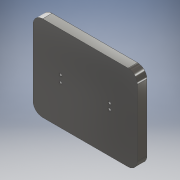
# Autodesk Inventor part: reverse gear stand
Saved by Autodesk Inventor 2017 (Build 210142000, 142)
## iProperties
Created: 2018-11-06
Part Number: reverse gear stand
Material: Generic
Document SubType Name: Modeling
Designer: User
Density: 1 g/cm^3
Appearance: Default
Author: User
Autodesk Inventor part; units mm, degrees
ref_plane "YZ Plane" through (0, 0, 0) normal (1, 0, 0) x (0, 1, 0)
ref_plane "XZ Plane" through (0, 0, 0) normal (0, 1, 0) x (-1, 0, 0)
ref_plane "XY Plane" through (0, 0, 0) normal (0, 0, 1) x (1, 0, 0)
sketch "Sketch2" plane through (0, 0, 0) normal (0, 1, 0) x (-1, 0, 0)
  line L0 (0, 0) -> (-220, 0)
  line L1 (-220, 0) -> (-220, -180)
  line L2 (-220, -180) -> (0, -180)
  line L3 (0, -180) -> (0, 0)
  dimension "d0" = 220
  dimension "d1" = 180
  constraints: 8 end point, 2 parallel, 1 horizontal, 1 perpendicular
  measures "d0" distance of L2.end L1.end
  measures "d1" distance of L1.end L0.end
extrude "Extrusion1" add sketch "Sketch2" along normal blind 20
sketch "Sketch3" plane through (0, 20, 0) normal (0, 1, 0) x (1, 0, 0)
  line L0 (0, 20) -> (0, 160)
  line L1 (0, 90) -> (46.5, 90)
  line L2 (46.5, 90) -> (173.5, 90)
  line L3 (173.5, 90) -> (173.5, 109)
  line L4 (173.5, 109) -> (173.5, 71)
  line L5 (173.5, 71) -> (46.5, 71)
  line L6 (46.5, 71) -> (46.5, 109)
  line L7 (46.5, 109) -> (173.5, 109)
  line L8 (0, 0) -> (220, 0) projected
  line L9 (220, 0) -> (220, 180) projected
  line L10 (220, 180) -> (0, 180) projected
  line L11 (0, 180) -> (0, 0) projected
  dimension "d4" = 46.5
  dimension "d5" = 127
  dimension "d6" = 19
  dimension "d7" = 38
  dimension "d11" = 71
  constraints: 16 end point, 4 perpendicular, 2 point on line, 1 horizontal, 1 midpoint
  measures "d4" distance of L1.start L1.end
  measures "d5" distance of L1.end L2.end
  measures "d6" distance of L2.end L3.end
  measures "d7" distance of L3.end L4.end
  measures "d11" distance between parallel lines of L10 L7
extrude "Extrusion2" cut sketch "Sketch3" against normal blind 10 contours L6 L7 L3 L2 | L2 L4 L5 L6
fillet "Fillet1" radius 20 4 edges at (0, 10, -180) (0, 10, 0) (220, 10, 0) (220, 10, -180)
fillet "Fillet2" radius 12 4 edges at (46.5, 15, -109) (173.5, 15, -109) (46.5, 15, -71) (173.5, 15, -71)
sketch "Sketch5" plane through (0, 0, 0) normal (0, -1, 0) x (1, 0, 0)
  line L0 (110, -90) -> (58.5, -90) construction
  line L1 (110, -90) -> (161.5, -90) construction
  line L2 (58.5, -90) -> (58.5, -97) construction
  line L3 (58.5, -97) -> (58.5, -83) construction
  line L4 (58.5, -83) -> (161.5, -83) construction
  line L5 (161.5, -83) -> (161.5, -97) construction
  circle A0 centre (58.5, -97) radius 2.5
  circle A1 centre (58.5, -83) radius 2.5
  circle A2 centre (161.5, -83) radius 2.5
  circle A3 centre (161.5, -94.5) radius 2.5
  line L6 (20, 0) -> (200, 0) projected
  arc A4 (200, -180) -> (220, -160) centre (200, -160) ccw projected
  line L7 (220, -20) -> (220, -160) projected
  arc A5 (220, -20) -> (200, 0) centre (200, -20) ccw projected
  line L8 (20, 0) -> (200, 0) projected
  arc A6 (20, 0) -> (0, -20) centre (20, -20) ccw projected
  line L9 (0, -160) -> (0, -20) projected
  arc A7 (0, -160) -> (20, -180) centre (20, -160) ccw projected
  line L10 (200, -180) -> (20, -180) projected
  point P0 (0, 0)
  point P1 (110, -90)
  dimension "d38" = 51.5
  dimension "d39" = 51.5
  dimension "d40" = 7
  dimension "d41" = 14
  dimension "d42" = 5
  dimension "d43" = 5
  dimension "d44" = 5
  dimension "d45" = 5
  dimension "d46" = 103
  dimension "d47" = 51.5
  dimension "d48" = 0
  dimension "d49" = 11.5
  dimension "d50" = 14
  dimension "d51" = 58.5
  dimension "d52" = 83
  constraints: 12 end point, 4 centre point, 3 coincident, 2 horizontal, 2 perpendicular, 2 point on line, 1 vertical
  measures "d38" distance of L0.start L0.end
  measures "d39" distance of L0.start L1.end
  measures "d40" distance of L0.end L2.end
  measures "d41" distance of L2.end L3.end
  measures "d42" diameter of A0
  measures "d43" diameter of A1
  measures "d44" diameter of A2
  measures "d45" diameter of A3
  measures "d46" distance between parallel lines of L2 L5
  measures "d47" distance from line of point (110, -90) L5
  measures "d48" distance from line of point (110, -90) L1
  measures "d49" distance from line of A3.centre L4
  measures "d50" distance from line of L5.end L4
  measures "d51" distance from line of L7 A3.centre
  measures "d52" distance from line of L10 L2.end
extrude "Extrusion4" cut sketch "Sketch5" against normal through all contours A0 | A1 | A2 | A3
body "Solid1"
